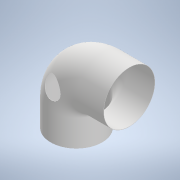
# Autodesk Inventor part: elbow
Saved by Autodesk Inventor 2021 (Build 250183000, 183)
## iProperties
Created: 2021-07-14
Part Number: elbow
Material: Generic
Document SubType Name: Modeling
Designer: HP
Density: 1 g/cm^3
Appearance: Default
Author: HP
Autodesk Inventor part; units mm, degrees
ref_plane "YZ Plane" through (0, 0, 0) normal (1, 0, 0) x (0, 1, 0)
ref_plane "XZ Plane" through (0, 0, 0) normal (0, 1, 0) x (-1, 0, 0)
ref_plane "XY Plane" through (0, 0, 0) normal (0, 0, 1) x (1, 0, 0)
sketch "Sketch1" plane through (0, 0, 0) normal (0, 0, 1) x (1, 0, 0)
  line L0 (0, 0) -> (0, 20)
  line L1 (20, 40) -> (40, 40)
  arc A0 (20, 40) -> (0, 20) centre (20, 20) ccw
  point P0 (0, 40)
  dimension "d0" = 40
  dimension "d1" = 40
  dimension "d2" = 20
  constraints: 4 end point, 2 point on circle, 2 point on line, 2 tangent, 1 centre point, 1 perpendicular, 1 vertical
  measures "d0" distance of L0.start point (0, 40)
  measures "d1" distance of point (0, 40) L1.end
  measures "d2" radius of A0
sketch "Sketch2" plane through (0, 0, 0) normal (0, 1, 0) x (-1, 0, 0)
  circle A0 centre (0, 0) radius 19.5
  circle A1 centre (0, 0) radius 19.25
  dimension "d3" = 39
  dimension "d4" = 38.5
  constraints: 2 centre point, 2 coincident
  measures "d3" diameter of A0
  measures "d4" diameter of A1
sweep "Sweep1" add profiles "Sketch2" path "Sketch1"
sketch "Sketch4" plane through (0, 0, 0) normal (0, 0, 1) x (1, 0, 0)
  circle A0 centre (0, 35.2694) radius 7.45
  point P0 (0, 0)
  dimension "d10" = 14.9
  constraints: 1 centre point
  measures "d10" diameter of A0
extrude "Extrusion2" cut sketch "Sketch4" against normal mid plane 40
body "Solid1"
